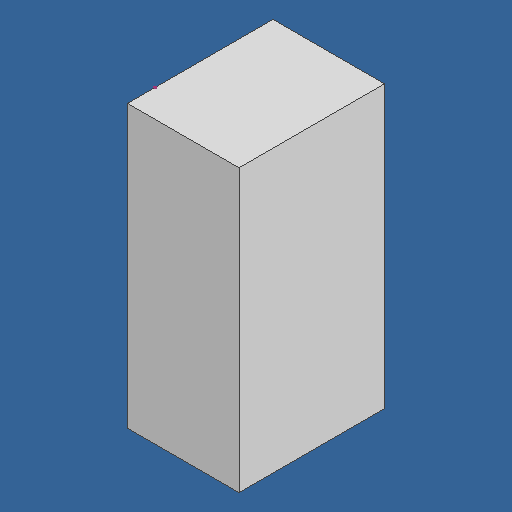
# Autodesk Inventor part: casing
Saved by Autodesk Inventor 2026.2 (Build 302298000, 298)
## iProperties
Created: 2026-01-15
Part Number: casing
Material: Generic
Document SubType Name: Modeling
Designer: Thoma
Density: 1 g/cm^3
Appearance: Default
Author: Thoma
Autodesk Inventor part; units mm, degrees
ref_plane "YZ Plane" through (0, 0, 0) normal (1, 0, 0) x (0, 1, 0)
ref_plane "XZ Plane" through (0, 0, 0) normal (0, 1, 0) x (-1, 0, 0)
ref_plane "XY Plane" through (0, 0, 0) normal (0, 0, 1) x (1, 0, 0)
sketch "Sketch1" plane through (0, 0, 0) normal (1, 0, 0) x (0, 1, 0)
  line L0 (40, 5.5916) -> (-18, 5.5916)
  line L1 (-18, 5.5916) -> (-18, -24.4084)
  line L2 (-18, -24.4084) -> (40, -24.4084)
  line L3 (40, -24.4084) -> (40, 5.5916)
  point P0 (0, 0)
  dimension "d0" = 58
  dimension "d1" = 30
  constraints: 8 end point, 2 parallel, 1 horizontal, 1 perpendicular
  measures "d0" distance of L1.end L2.end
  measures "d1" distance of L2.end L0.start
extrude "Extrusion1" add sketch "Sketch1" along normal blind 23
sketch "Sketch2" plane through (0, 40, 5.5916) normal (0, 1, 0) x (1, 0, 0)
  point P0 (0, 5.5916)
body "Solid1"
